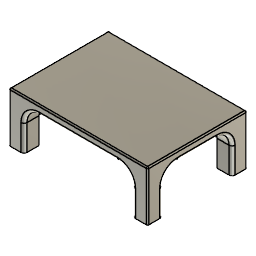
Box_V2 (Autodesk Fusion 360 design; units mm, degrees)
Autodesk Fusion 360 part; units mm, degrees
sketch "Boceto1" plane through (0, 0, 0) normal (0, 0, 1) x (1, 0, 0)
  line L0 (0, 0) -> (230, 0)
  line L1 (230, 0) -> (230, 165)
  line L2 (230, 165) -> (0, 165)
  line L3 (0, 165) -> (0, 0)
  line L4 (0, 165) -> (25, 165)
  line L5 (25, 165) -> (25, 140)
  line L6 (25, 140) -> (0, 140)
  line L7 (0, 140) -> (0, 165)
  line L8 (230, 165) -> (205, 165)
  line L9 (205, 165) -> (205, 140)
  line L10 (205, 140) -> (230, 140)
  line L11 (230, 140) -> (230, 165)
  line L12 (230, 0) -> (205, 0)
  line L13 (205, 0) -> (205, 25)
  line L14 (205, 25) -> (230, 25)
  line L15 (230, 25) -> (230, 0)
  line L16 (0, 0) -> (25, 0)
  line L17 (25, 0) -> (25, 25)
  line L18 (25, 25) -> (0, 25)
  line L19 (0, 25) -> (0, 0)
  dimension "d1" = 230
  dimension "d2" = 165
  dimension "d12" = 25
  constraint horizontal L0
  constraint vertical L1
  constraint horizontal L2
  constraint vertical L3
  constraint coincident L0.start L3.end
  constraint horizontal L4
  constraint vertical L5
  constraint horizontal L6
  constraint vertical L7
  constraint equal L5 L6
  constraint horizontal L8
  constraint vertical L9
  constraint horizontal L10
  constraint vertical L11
  constraint horizontal L12
  constraint vertical L13
  constraint horizontal L14
  constraint vertical L15
  constraint horizontal L16
  constraint vertical L17
  constraint horizontal L18
  constraint vertical L19
  constraint equal L6 L18
  constraint equal L6 L10
  constraint equal L6 L14
  constraint equal L13 L14
  constraint equal L9 L10
  constraint equal L17 L18
  measures "d1" distance of L0.start L0.end
  measures "d2" distance of L0.start L2.end
  measures "d12" distance of L2.end L6.end
ref_plane "WorkPlane1" through (115, 82.5, 83) normal (0, 0, 1) x (1, 0, 0)
extrude "Extrude4" add sketch "Boceto1" along normal blind 83 contours L0 L3 L16 L17 L18 L19 | L0 L1 L12 L13 L14 L15 | L2 L3 L4 L5 L6 L7 | L1 L2 L8 L9 L10 L11 makes body 1 at (0, 16.6667, 27.6667) makes body 2 at (205, 8.3333, 27.6667) makes body 3 at (0, 156.6667, 27.6667) makes body 4 at (213.3333, 140, 27.6667)
sketch "Sketch4" plane through (0, 0, 83) normal (0, 0, 1) x (1, 0, 0)
  line L0 (25, 25) -> (0, 25)
  line L1 (25, 0) -> (25, 25)
  line L2 (0, 0) -> (25, 0)
  line L3 (0, 25) -> (0, 0)
  line L4 (0, 140) -> (0, 165)
  line L5 (0, 165) -> (25, 165)
  line L6 (25, 165) -> (25, 140)
  line L7 (25, 140) -> (0, 140)
  line L8 (205, 140) -> (230, 140)
  line L9 (205, 165) -> (205, 140)
  line L10 (230, 165) -> (205, 165)
  line L11 (230, 140) -> (230, 165)
  line L12 (230, 25) -> (230, 0)
  line L13 (230, 0) -> (205, 0)
  line L14 (205, 0) -> (205, 25)
  line L15 (205, 25) -> (230, 25)
  line L16 (0, 0) -> (230, 0)
  line L17 (230, 0) -> (230, 165)
  line L18 (230, 165) -> (0, 165)
  line L19 (0, 165) -> (0, 0)
  constraint horizontal L16
  constraint vertical L17
  constraint horizontal L18
  constraint vertical L19
  constraint coincident L10.start L11.end
  constraint coincident L2.start L3.end
extrude "Extrude5" add sketch "Sketch4" against normal blind 15 bodies 1 2 3 4
sketch "Sketch5" plane through (0, 0, 83) normal (0, 0, 1) x (-1, 0, 0)
  line L0 (-230, -165) -> (0, -165)
  line L1 (0, -165) -> (0, 0)
  line L2 (0, 0) -> (-230, 0)
  line L3 (-230, 0) -> (-230, -165)
  line L4 (-5, -5) -> (-225, -5)
  line L5 (-225, -5) -> (-225, -160)
  line L6 (-225, -160) -> (-5, -160)
  line L7 (-5, -160) -> (-5, -5)
  dimension "d17" = -5
fillet "Fillet1" radius 25 8 edges at (12.5, 25, 68) (25, 12.5, 68) (25, 152.5, 68) (12.5, 140, 68) (217.5, 140, 68) (205, 152.5, 68) (205, 12.5, 68) (217.5, 25, 68) on bodies 1
fillet "Fillet2" radius 5 20 edges at (205, 0, 21.5) (197.6777, 0, 60.6777) (115, 0, 68) (32.3223, 0, 60.6777) (25, 0, 21.5) (230, 140, 21.5) (230, 132.6777, 60.6777) (230, 82.5, 68) (230, 32.3223, 60.6777) (230, 25, 21.5) (25, 165, 21.5) (32.3223, 165, 60.6777) (115, 165, 68) (197.6777, 165, 60.6777) (205, 165, 21.5) (0, 25, 21.5) (0, 32.3223, 60.6777) (0, 82.5, 68) (0, 132.6777, 60.6777) (0, 140, 21.5) on bodies 1
fillet "Fillet3" radius 2 8 edges at (0, 82.5, 83) (115, 0, 83) (0, 0, 41.5) (230, 0, 41.5) (230, 82.5, 83) (230, 165, 41.5) (115, 165, 83) (0, 165, 41.5) on bodies 1
